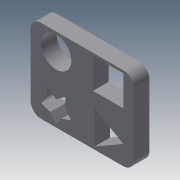
# Autodesk Inventor part: PassengerBase
Saved by Autodesk Inventor 2015 (Build 190159000, 159)
## iProperties
Created: 2016-11-04
Part Number: PassengerBase
Material: Generic
Document SubType Name: Modeling
Designer: Aniket Pant
Density: 1 g/cm^3
Appearance: Default
Author: Aniket Pant
Autodesk Inventor part; units mm, degrees
ref_plane "YZ Plane" through (0, 0, 0) normal (1, 0, 0) x (0, 1, 0)
ref_plane "XZ Plane" through (0, 0, 0) normal (0, 1, 0) x (-1, 0, 0)
ref_plane "XY Plane" through (0, 0, 0) normal (0, 0, 1) x (1, 0, 0)
sketch "Sketch1" plane through (0, 0, 0) normal (0, 0, 1) x (1, 0, 0)
  line L0 (5.08, 0) -> (45.085, 0)
  line L1 (50.165, 5.08) -> (50.165, 35.306)
  line L2 (45.085, 40.386) -> (5.08, 40.386)
  line L3 (0, 35.306) -> (0, 5.08)
  arc A0 (5.08, 40.386) -> (0, 35.306) centre (5.08, 35.306) ccw
  arc A1 (50.165, 35.306) -> (45.085, 40.386) centre (45.085, 35.306) ccw
  arc A2 (45.085, 0) -> (50.165, 5.08) centre (45.085, 5.08) ccw
  arc A3 (0, 5.08) -> (5.08, 0) centre (5.08, 5.08) ccw
  circle A4 centre (12.446, 31.75) radius 7.366
  line L4 (30.353, 39.116) -> (45.085, 39.116)
  line L5 (45.085, 39.116) -> (45.085, 24.384)
  line L6 (45.085, 24.384) -> (30.353, 24.384)
  line L7 (30.353, 24.384) -> (30.353, 39.116)
  line L8 (31.0509, 17.4752) -> (45.085, 9.3726)
  line L9 (45.085, 9.3726) -> (31.0509, 1.27)
  line L10 (31.0509, 1.27) -> (31.0509, 17.4752)
  circle A5 centre (12.3952, 8.9553) radius 7.6853 construction
  line L11 (12.3952, 1.27) -> (5.086, 6.5804) construction
  line L12 (5.086, 6.5804) -> (7.8779, 15.1729) construction
  line L13 (7.8779, 15.1729) -> (16.9125, 15.1729) construction
  line L14 (16.9125, 15.1729) -> (19.7044, 6.5804) construction
  line L15 (19.7044, 6.5804) -> (12.3952, 1.27) construction
  line L16 (7.8779, 15.1729) -> (7.8779, 10.4231)
  line L17 (7.8779, 10.4231) -> (5.086, 6.5804)
  line L18 (5.086, 6.5804) -> (9.6033, 5.1127)
  line L19 (9.6033, 5.1127) -> (12.3952, 1.27)
  line L20 (12.3952, 1.27) -> (15.1871, 5.1127)
  line L21 (15.1871, 5.1127) -> (19.7044, 6.5804)
  line L22 (19.7044, 6.5804) -> (16.9125, 10.4231)
  line L23 (16.9125, 10.4231) -> (16.9125, 15.1729)
  line L24 (16.9125, 15.1729) -> (12.3952, 11.8909)
  line L25 (12.3952, 11.8909) -> (7.8779, 15.1729)
  point P0 (0, 0)
  point P1 (50.165, 40.386)
  point P2 (50.165, 0)
  point P3 (0, 40.386)
  point P4 (35.7289, 9.3726)
  dimension "d0" = 50.165
  dimension "d1" = 40.386
  dimension "d2" = 5.08
  dimension "d3" = 14.732
  dimension "d4" = 12.446
  dimension "d5" = 8.636
  dimension "d6" = 14.732
  dimension "d7" = 14.732
  dimension "d8" = 1.27
  dimension "d9" = 5.08
  dimension "d20" = 16.2052
  dimension "d21" = 1.27
  dimension "d22" = 5.08
  dimension "d23" = 4.7498
  dimension "d24" = 4.7498
  dimension "d25" = 2.3749
  dimension "d26" = 12.3952
  dimension "d27" = 1.27
  constraints: 52 end point, 8 point on circle, 8 point on line, 8 tangent, 5 centre point, 5 equal length, 5 parallel, 4 perpendicular, 3 equal radius, 2 horizontal, 2 vertical, 1 coincident, 1 vertical alignment, 20 other
  measures "d0" distance of point (50.165, 40.386) point (0, 40.386)
  measures "d1" distance of point (50.165, 0) point (50.165, 40.386)
  measures "d2" radius of A0
  measures "d3" diameter of A4
  measures "d4" distance from line of L3 A4.centre
  measures "d5" distance from line of L2 A4.centre
  measures "d6" distance of L4.start L4.end
  measures "d7" distance of L4.end L5.end
  measures "d8" distance between parallel lines of L2 L4
  measures "d9" distance between parallel lines of L1 L5
  measures "d20" distance of L9.end L8.start
  measures "d21" distance from line of L0 L9.end
  measures "d22" distance from line of L1 L8.end
  measures "d23" distance of L12.end L16.end
  measures "d24" distance of L22.end L13.end
  measures "d25" vertical distance of L14.end point (12.395, 8.955)
  measures "d26" distance from line of L3 L11.start
  measures "d27" distance from line of L0 L11.start
extrude "Extrusion1" add sketch "Sketch1" along normal blind 7.62
body "Solid1"
